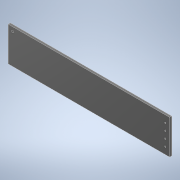
# Autodesk Inventor part: Tabla_movimiento
Saved by Autodesk Inventor 2022 (Build 260153000, 153)
## iProperties
Created: 2023-04-08
Part Number: Tabla_movimiento
Material: Plástico ABS
Document SubType Name: Modeling
Designer: USUARIO
Density: 1.06 g/cm^3
Appearance: Suave - Negro
Author: USUARIO
Autodesk Inventor part; units mm, degrees
ref_plane "YZ Plane" through (0, 0, 0) normal (1, 0, 0) x (0, 1, 0)
ref_plane "XZ Plane" through (0, 0, 0) normal (0, 1, 0) x (-1, 0, 0)
ref_plane "XY Plane" through (0, 0, 0) normal (0, 0, 1) x (1, 0, 0)
sketch "Boceto1" plane through (0, 0, 0) normal (0, 0, 1) x (1, 0, 0)
  line L0 (0, 0) -> (750, 0)
  line L1 (750, 0) -> (750, -160)
  line L2 (750, -160) -> (0, -160)
  line L3 (0, -160) -> (0, 0)
  dimension "d0" = 750
  dimension "d1" = 160
  constraints: 8 end point, 2 parallel, 1 horizontal, 1 perpendicular
  measures "d0" distance of L1.end L2.end
  measures "d1" distance of L0.end L1.end
extrude "Extrusión1" add sketch "Boceto1" along normal blind 10
sketch "Boceto2" plane through (0, 0, 10) normal (0, 0, 1) x (1, 0, 0)
  line L0 (750, 0) -> (0, 0) projected
  line L1 (0, 0) -> (40, 0)
  line L2 (40, 0) -> (40, -40)
  line L3 (40, -40) -> (0, -40)
  line L4 (0, -40) -> (0, 0)
  circle A0 centre (20, -20) radius 5
  dimension "d4" = 40
  dimension "d5" = 40
  dimension "d6" = 10
  constraints: 8 end point, 2 parallel, 1 centre point, 1 horizontal, 1 perpendicular
  measures "d4" distance of L2.end L3.end
  measures "d5" distance of L1.end L2.end
  measures "d6" diameter of A0
extrude "Extrusión2" cut sketch "Boceto2" against normal blind 10 contours A0
sketch "Boceto4" plane through (0, 0, 10) normal (0, 0, 1) x (1, 0, 0)
  line L0 (0, -160) -> (750, -160) projected
  line L1 (750, -160) -> (730, -160)
  line L2 (730, -160) -> (730, -128)
  line L3 (730, -128) -> (730, -96)
  line L4 (730, -96) -> (730, -64)
  line L5 (730, -64) -> (730, -32)
  circle A0 centre (730, -128) radius 3
  circle A1 centre (730, -96) radius 3
  circle A2 centre (730, -64) radius 3
  circle A3 centre (730, -32) radius 3
  point P0 (0, 0)
  dimension "d13" = 20
  dimension "d14" = 32
  dimension "d15" = 32
  dimension "d16" = 32
  dimension "d17" = 32
  dimension "d18" = 6
  dimension "d19" = 6
  dimension "d20" = 6
  dimension "d21" = 6
  constraints: 10 end point, 4 centre point, 4 coincident, 4 point on line, 1 perpendicular
  measures "d13" distance of L0.end L1.end
  measures "d14" distance of L1.end L2.end
  measures "d15" distance of L2.end L3.end
  measures "d16" distance of L3.end L4.end
  measures "d17" distance of L4.end L5.end
  measures "d18" diameter of A0
  measures "d19" diameter of A1
  measures "d20" diameter of A2
  measures "d21" diameter of A3
extrude "Extrusión4" cut sketch "Boceto4" against normal blind 10
